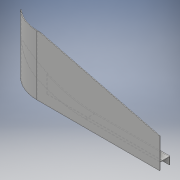
# Autodesk Inventor part: endplate_ver2
Saved by Autodesk Inventor 2018 (Build 220112000, 112)
## iProperties
Created: 2018-05-11
Part Number: endplate_ver2
Material: 一般
Document SubType Name: Modeling
Designer: ku_sk
Density: 1 g/cm^3
Appearance: 既定
Author: ku_sk
Autodesk Inventor part; units mm, degrees
ref_plane "YZ Plane" through (0, 0, 0) normal (1, 0, 0) x (0, 1, 0)
ref_plane "XZ Plane" through (0, 0, 0) normal (0, 1, 0) x (-1, 0, 0)
ref_plane "XY Plane" through (0, 0, 0) normal (0, 0, 1) x (1, 0, 0)
sketch "スケッチ1" plane through (0, 0, 0) normal (0, 1, 0) x (-1, 0, 0)
  line L0 (250, 100) -> (-250, 100)
  line L1 (-250, 100) -> (-250, -100)
  line L2 (-250, -100) -> (250, -100)
  line L3 (250, -100) -> (250, 100)
  point P0 (0, 0)
  dimension "d2" = 250
  dimension "d3" = 500
  dimension "d4" = 100
  dimension "d5" = 200
  constraints: 8 end point, 2 parallel, 1 horizontal, 1 perpendicular
  measures "d2" distance from line of point (0, 0) L3
  measures "d3" distance of L0.start L0.end
  measures "d4" distance from line of point (0, 0) L0
  measures "d5" distance of L2.end L0.start
extrude "押し出し1" add sketch "スケッチ1" along normal blind 35
sketch "スケッチ2" plane through (-250, 0, 100) normal (0, 0, 1) x (1, 0, 0)
  line L0 (0, 35) -> (500, 35) projected
  line L1 (0, 0) -> (500, 0) projected
  arc A0 (0, 35) -> (90, 0) centre (90, 133.2143) ccw
  line L2 (0, 0) -> (0, 35) projected
  point P0 (250, 0)
  dimension "d8" = 90
  constraints: 2 point on circle, 1 centre point, 1 point on line, 1 tangent
  measures "d8" distance from line of L2 A0.end
extrude "押し出し2" cut sketch "スケッチ2" against normal through all
sketch "スケッチ5" plane through (-160, 0, 100) normal (0, 0, 1) x (1, 0, 0)
  arc A0 (-90, 35) -> (0, 0) centre (0, 133.2143) ccw projected
  line L0 (0, 0) -> (410, 0) projected
  arc A1 (-87.0123, 35) -> (0, 2) centre (0, 133.2143) ccw
  line L1 (0, 2) -> (54.4195, 2)
  line L2 (54.4195, 2) -> (410, 2)
  line L3 (-90, 35) -> (410, 35) projected
  line L4 (410, 0) -> (410, 35) projected
  point P0 (160, 0)
  point P1 (40, 35)
  dimension "d20" = 2
  constraints: 4 end point, 2 point on circle, 1 centre point, 1 collinear, 1 point on line, 1 other
  measures "d20" radial gap between concentric circles of A0 A1
extrude "押し出し5" cut sketch "スケッチ5" against normal through all contours L3 L4 L2 L1 A1
sketch "スケッチ8" plane through (-160, 2, 100) normal (0, 1, 0) x (1, 0, 0)
  line L0 (410, 175) -> (160, 175)
  line L1 (410, 200) -> (410, 0) projected
  line L2 (0, 200) -> (410, 200) projected
  arc A0 (160, 175) -> (-90, 80) centre (160, -201.4474) ccw
  line L3 (-90, 200) -> (-90, 0) projected
  line L4 (-87.0123, 200) -> (0, 200) projected
  line L5 (-87.0123, 200) -> (-90, 200) projected
  line L6 (410, 177) -> (160, 177)
  arc A1 (160, 177) -> (-90, 82.6695) centre (160, -201.4474) ccw
  line L7 (410, 175) -> (410, 177)
  line L8 (410, 0) -> (410, 200) projected
  line L9 (-90, 82.6695) -> (-90, 80)
  point P0 (160, 100)
  dimension "d35" = 25
  dimension "d36" = 120
  dimension "d37" = 250
  dimension "d38" = 2
  constraints: 8 end point, 4 point on circle, 3 point on line, 2 centre point, 1 collinear, 1 horizontal, 1 parallel, 1 tangent, 1 other
  measures "d35" distance between parallel lines of L2 L0
  measures "d36" distance from line of L9.end L2
  measures "d37" distance of L0.start L0.end
  measures "d38" distance between parallel lines of L0 L6
extrude "押し出し7" add sketch "スケッチ8" along normal up to surface (33 mm away) contours L0 A0 L3 A1 L6 L1
delete faces "面を削除1" heal yes whole lump no faces at (-239.2435, 9.8792, 10.8013) (-250, 13, 18.2203) (-242.947, 2, 13.2909) (-239.2361, 9.8796, 8.2094)
sketch "スケッチ9" plane through (0, 35, -75) normal (0, 1, 0) x (1, 0, 0)
  line L0 (250, 25) -> (250, 2) projected
  line L1 (0, 2) -> (250, 2) projected
  line L2 (250, 25) -> (250, 2) projected
  line L3 (-160, 25) -> (250, 25) projected
  line L4 (-160, -33.4861) -> (-160, 25) projected
  arc A0 (0, 2) -> (-160, -33.4861) centre (0, -376.4474) ccw projected
  point P0 (0, -75)
extrude "押し出し8" add sketch "スケッチ9" against normal blind 2
sketch "スケッチ10" plane through (-160, 2, 100) normal (0, 1, 0) x (1, 0, 0)
  line L0 (410, 175) -> (410, 0) projected
  line L1 (410, 0) -> (0, 0) projected
  line L2 (410, 0) -> (410, 200) projected
  line L3 (410, 100) -> (10, 0)
  line L4 (0, 0) -> (410, 0) projected
  point P0 (160, 100)
  dimension "d43" = 400
  dimension "d44" = 100
  constraints: 3 point on line, 2 end point, 1 midpoint
  measures "d43" distance from line of L0 L3.end
  measures "d44" distance from line of L3.start L1
extrude "押し出し9" cut sketch "スケッチ10" against normal through all
